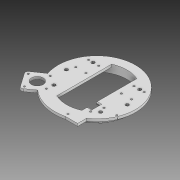
# Autodesk Inventor part: SwivelMount
Saved by Autodesk Inventor 2020 (Build 240168000, 168)
## iProperties
Created: 2020-09-15
Part Number: SwivelMount
Material: Generic
Document SubType Name: Modeling
Designer: DDeGo
Density: 1 g/cm^3
Appearance: Default
Author: DDeGo
Autodesk Inventor part; units mm, degrees
ref_plane "YZ Plane" through (0, 0, 0) normal (1, 0, 0) x (0, 1, 0)
ref_plane "XZ Plane" through (0, 0, 0) normal (0, 1, 0) x (-1, 0, 0)
ref_plane "XY Plane" through (0, 0, 0) normal (0, 0, 1) x (1, 0, 0)
sketch "Sketch1" plane through (0, 0, 0) normal (1, 0, 0) x (0, 1, 0)
  line L0 (0, 0) -> (0, -59.4) construction
  line L1 (0, -59.4) -> (7.5, -59.4)
  line L2 (7.5, -59.4) -> (7.5, -66.4) construction
  line L3 (7.5, -66.4) -> (5, -66.4)
  line L4 (5, -66.4) -> (5, -63.4)
  line L5 (5, -63.4) -> (0, -63.4)
  line L6 (0, -63.4) -> (0, -59.4)
  line L7 (0, 0) -> (7.5, 0) construction
  line L8 (7.5, 0) -> (7.5, -66.4) construction
  line L9 (7.5, -66.4) -> (11, -66.4)
  line L10 (11, -66.4) -> (11, -76)
  line L11 (11, -76) -> (16, -76)
  line L12 (16, -76) -> (16, -59.4)
  line L13 (16, -59.4) -> (7.5, -59.4)
  dimension "d0" = 63.4
  dimension "d1" = 4
  dimension "d2" = 2.5
  dimension "d3" = 3
  dimension "d4" = 5
  dimension "d6" = 6
  dimension "d7" = 5
  dimension "d8" = 76
  constraints: 28 end point, 10 perpendicular, 2 horizontal, 1 collinear, 1 point on line, 1 vertical
  measures "d0" distance from line of L0.start L5
  measures "d1" distance between parallel lines of L1 L5
  measures "d2" distance between parallel lines of L2 L4
  measures "d3" distance of L3.end L4.end
  measures "d4" distance of L4.end L5.end
  measures "d6" distance between parallel lines of L4 L10
  measures "d7" distance of L10.end L11.end
  measures "d8" distance between parallel lines of L7 L11
revolve "Revolution1" add sketch "Sketch1" angle 360 about axis through (0, 0, 0) along (0, 1, 0)
sketch "Sketch2" plane through (0, 16, 0) normal (0, 1, 0) x (1, 0, 0)
  line L0 (-24.75, -59.4) -> (24.75, -59.4)
  line L1 (24.75, -59.4) -> (24.75, 59.4)
  line L2 (24.75, 59.4) -> (-24.75, 59.4)
  line L3 (-24.75, 59.4) -> (-24.75, -59.4)
  line L4 (-24.75, -59.4) -> (24.75, 59.4) construction
  line L5 (24.75, -59.4) -> (-24.75, 59.4) construction
  circle A0 centre (0, 0) radius 59.4 projected
  point P0 (24.75, -53.9981)
  point P1 (24.75, 53.9981)
  point P2 (-24.75, -53.9981)
  point P3 (-24.75, 53.9981)
  dimension "d9" = 49.5
  constraints: 12 end point, 2 midpoint, 2 parallel, 1 horizontal, 1 perpendicular, 1 tangent
  measures "d9" distance of L1.end L2.end
extrude "Extrusion1" add sketch "Sketch2" against normal blind 5 contours A0 L3 | L1 A0
sketch "Sketch3" plane through (0, 16, 0) normal (0, 1, 0) x (1, 0, 0)
  line L0 (-44.75, 26) -> (0, 26) construction
  line L1 (24.75, 53.9981) -> (24.75, -53.9981) projected
  line L2 (-24.75, -53.9981) -> (-24.75, 53.9981) projected
  line L3 (-34.75, 13.5) -> (-54.75, 13.5) construction
  line L4 (-54.75, 13.5) -> (-54.75, 38.5) construction
  line L5 (-54.75, 38.5) -> (-34.75, 38.5) construction
  line L6 (-34.75, 38.5) -> (-34.75, 13.5) construction
  line L7 (-34.75, 13.5) -> (-54.75, 38.5) construction
  line L8 (-54.75, 13.5) -> (-34.75, 38.5) construction
  line L9 (0, 0) -> (0, 26) construction
  circle A0 centre (-54.75, 13.5) radius 1.75
  circle A1 centre (-54.75, 38.5) radius 1.75
  circle A2 centre (-34.75, 38.5) radius 1.75
  circle A3 centre (-34.75, 13.5) radius 1.75
  line L10 (34.75, 13.5) -> (54.75, 13.5) construction
  line L11 (54.75, 13.5) -> (54.75, 38.5) construction
  line L12 (54.75, 38.5) -> (34.75, 38.5) construction
  line L13 (34.75, 38.5) -> (34.75, 13.5) construction
  line L14 (34.75, 13.5) -> (54.75, 38.5) construction
  line L15 (54.75, 13.5) -> (34.75, 38.5) construction
  circle A4 centre (54.75, 13.5) radius 1.75
  circle A5 centre (54.75, 38.5) radius 1.75
  circle A6 centre (34.75, 38.5) radius 1.75
  circle A7 centre (34.75, 13.5) radius 1.75
  point P0 (44.75, 26)
  dimension "d12" = 26
  dimension "d14" = 20
  dimension "d15" = 25
  dimension "d16" = 20
  dimension "d17" = 3.5
  constraints: 28 end point, 9 symmetric about line, 8 centre point, 8 coincident, 4 midpoint, 3 equal radius, 2 horizontal, 2 parallel, 1 perpendicular, 1 vertical, 4 other
  measures "d12" distance from line of L9.start L0
  measures "d14" distance from line of L0.start L2
  measures "d15" distance of L3.end L4.end
  measures "d16" distance of L4.end L5.end
  measures "d17" diameter of A0
extrude "Extrusion2" cut sketch "Sketch3" against normal through all
sketch "Sketch4" plane through (0, 16, 0) normal (0, 1, 0) x (1, 0, 0)
  circle A0 centre (0, 0) radius 76 projected
  line L0 (25, -131.7705) -> (-25, -131.7705)
  line L1 (-25, -131.7705) -> (-25, -71.7705)
  line L2 (-25, -71.7705) -> (25, -71.7705) construction
  line L3 (25, -71.7705) -> (25, -131.7705)
  line L4 (25, -131.7705) -> (-25, -71.7705) construction
  line L5 (-25, -131.7705) -> (25, -71.7705) construction
  line L6 (0, -101.7705) -> (0, 0) construction
  point P0 (0, 0)
  dimension "d20" = 60
  dimension "d21" = 50
  constraints: 14 end point, 2 midpoint, 2 parallel, 1 horizontal, 1 perpendicular, 1 vertical, 2 other
  measures "d20" distance of L0.end L1.end
  measures "d21" distance of L0.start L0.end
extrude "Extrusion3" add sketch "Sketch4" against normal up to surface (5 mm away) contours A0 L3 L0 L1
sketch "Sketch5" plane through (-25, 16, 131.7705) normal (0, 1, 0) x (1, 0, 0)
  line L0 (-38.6517, 112.8373) -> (-14.5615, 78.433)
  line L1 (-14.5615, 78.433) -> (-44.8701, 57.2106)
  line L2 (-51.8337, 58.4385) -> (-70.1882, 84.6514)
  line L3 (-68.9603, 91.615) -> (-38.6517, 112.8373)
  line L4 (-22.2215, 79.7836) -> (-40.0023, 105.1773) construction
  line L5 (-40.0023, 105.1773) -> (-65.3961, 87.3965) construction
  line L6 (-65.3961, 87.3965) -> (-47.6152, 62.0028) construction
  line L7 (-47.6152, 62.0028) -> (-22.2215, 79.7836) construction
  arc A0 (50, 60) -> (0, 60) centre (25, 131.7705) ccw projected
  line L8 (-65.3961, 87.3965) -> (-22.2215, 79.7836) construction
  circle A1 centre (25, 131.7705) radius 63.4 projected
  line L9 (-43.8088, 83.59) -> (-26.9342, 95.4057) construction
  line L10 (-26.9342, 95.4057) -> (25, 131.7705) construction
  circle A2 centre (-40.0023, 105.1773) radius 1.75
  circle A3 centre (-65.3961, 87.3965) radius 1.75
  circle A4 centre (-43.8088, 83.59) radius 11.5
  circle A5 centre (-47.6152, 62.0028) radius 1.75
  circle A6 centre (-22.2215, 79.7836) radius 1.75
  line L11 (25, 131.7705) -> (25, 92.5102) construction
  arc A7 (-68.9603, 91.615) -> (-70.1882, 84.6514) centre (-66.0924, 87.5193) ccw
  arc A8 (-51.8337, 58.4385) -> (-44.8701, 57.2106) centre (-47.738, 61.3064) ccw
  point P0 (-48.9659, 54.3427)
  point P1 (-73.0561, 88.7471)
  point P2 (-22.7866, 72.6736)
  point P3 (-46.8769, 107.078)
  dimension "d24" = 20.6
  dimension "d25" = 31
  dimension "d26" = 42
  dimension "d29" = 3.5
  dimension "d30" = 23
  dimension "d31" = 55
  dimension "d37" = 5
  dimension "d38" = 84
  constraints: 24 end point, 7 centre point, 5 coincident, 4 equal radius, 4 parallel, 4 perpendicular, 4 point on circle, 4 point on line, 4 tangent, 1 collinear, 1 midpoint, 1 vertical, 5 other
  measures "d24" distance of L9.start L9.end
  measures "d25" distance of L5.end L6.end
  measures "d26" distance of point (-48.966, 54.343) point (-73.056, 88.747)
  measures "d29" diameter of A6
  measures "d30" diameter of A4
  measures "d31" angle of L10 L11
  measures "d37" radius of A7
  measures "d38" distance of point (25, 131.77) A4.centre
extrude "Extrusion4" add sketch "Sketch5" against normal up to surface (5 mm away) contours L0 A1 L1 A0 A4 L3 | L0 A1 | A0 A4 L1 A8 L2 A7 L3 | A4 A0 | A0 A4 | A2 | A3 | A5 | A6 picked at (-26.2496, 94.9188)
extrude "Extrusion5" cut sketch "Sketch5" against normal through all contours A4 A0 | A0 A4 | A2 | A3 | A5 | A6
sketch "Sketch6" plane through (-25, 11, 131.7705) normal (0, -1, 0) x (1, 0, 0)
  circle A0 centre (-65.3961, -87.3965) radius 1.75 projected
  circle A1 centre (-65.3961, -87.3965) radius 3
  circle A2 centre (-47.6152, -62.0028) radius 1.75 projected
  circle A3 centre (-47.6152, -62.0028) radius 3
  circle A4 centre (-22.2215, -79.7836) radius 1.75 projected
  circle A5 centre (-22.2215, -79.7836) radius 3
  circle A6 centre (-40.0023, -105.1773) radius 1.75 projected
  circle A7 centre (-40.0023, -105.1773) radius 3
  point P0 (25, -131.7705)
  dimension "d34" = 6
  constraints: 4 centre point, 4 coincident, 3 equal radius
  measures "d34" diameter of A1
extrude "Extrusion6" cut sketch "Sketch6" against normal blind 3 contours A0 | A1 | A2 | A3 | A4 | A5 | A6 | A7
ref_plane "Work Plane1" through (38.75, 16, -53.9981) normal (-1, 0, 0) x (0, 0, 1)
sketch "Sketch7" plane through (38.75, 16, -53.9981) normal (-1, 0, 0) x (0, 0, 1)
  line L0 (13.7481, 0) -> (17.2481, 0) projected
  line L1 (38.7481, 0) -> (42.2481, 0) projected
  line L2 (15.4981, 0) -> (27.9981, 40) construction
  line L3 (27.9981, 40) -> (40.4981, 0) construction
  line L4 (27.9981, 40) -> (109.9356, 21.5) construction
  line L5 (94.4356, 37) -> (125.4356, 37) construction
  line L6 (125.4356, 37) -> (125.4356, 6) construction
  line L7 (125.4356, 6) -> (94.4356, 6) construction
  line L8 (94.4356, 6) -> (94.4356, 37) construction
  line L9 (94.4356, 37) -> (125.4356, 6) construction
  line L10 (125.4356, 37) -> (94.4356, 6) construction
  circle A0 centre (109.9356, 21.5) radius 11.5
  circle A1 centre (125.4356, 37) radius 1.75
  circle A2 centre (125.4356, 6) radius 1.75
  circle A3 centre (94.4356, 6) radius 1.75
  circle A4 centre (94.4356, 37) radius 1.75
  line L11 (88.4356, 0) -> (131.4356, 0)
  line L12 (131.4356, 0) -> (131.4356, 43)
  line L13 (131.4356, 43) -> (88.4356, 43)
  line L14 (88.4356, 43) -> (88.4356, 0)
  line L15 (88.4356, 0) -> (131.4356, 43) construction
  line L16 (131.4356, 0) -> (88.4356, 43) construction
  line L17 (0, 0) -> (107.9962, 0) projected
  point P0 (53.9981, -16)
  dimension "d40" = 84
  dimension "d41" = 23
  dimension "d42" = 3.5
  dimension "d43" = 31
  dimension "d44" = 31
  dimension "d46" = 40
  dimension "d47" = 43
  dimension "d84" = 81.9375
  constraints: 30 end point, 6 midpoint, 5 centre point, 5 coincident, 4 parallel, 3 equal radius, 2 horizontal, 2 perpendicular, 1 equal length, 1 point on line, 2 other
  measures "d40" distance of L2.end L4.end
  measures "d41" diameter of A0
  measures "d42" diameter of A4
  measures "d43" distance of L5.start L5.end
  measures "d44" distance of L7.end L5.start
  measures "d46" distance from line of L1 L2.end
  measures "d47" distance of L11.end L12.end
  measures "d84" horizontal distance of L4.end L2.end
extrude "Extrusion7" add sketch "Sketch7" against normal blind 4
sketch "Sketch8" plane through (38.75, 16, 65.3792) normal (0, -1, 0) x (1, 0, 0)
  arc A0 (-110.6269, -40.6867) -> (4, -2.5426) centre (-38.75, -65.3792) ccw projected
  line L0 (0, 12.0583) -> (4, 12.0583) projected
  line L1 (4, -2.5426) -> (4, 12.0583)
  line L2 (4, 12.0583) -> (-13.75, 12.0583)
  line L3 (-13.75, 66.3913) -> (-13.75, 6.3913) projected
  arc A1 (0, 0) -> (-13.75, 6.3913) centre (-38.75, -65.3792) ccw projected
  line L4 (-13.75, 12.0583) -> (-13.75, 6.3913)
  arc A2 (4, -2.5426) -> (-13.75, 6.3913) centre (-38.75, -65.3792) ccw
  arc A3 (-110.6269, -40.6867) -> (-13.75, 6.3913) centre (-38.75, -65.3792) ccw projected
  constraints: 6 end point, 2 perpendicular, 2 point on circle, 1 centre point, 1 concentric, 1 point on line, 1 vertical
extrude "Extrusion8" add sketch "Sketch8" along normal up to surface (5 mm away)
sketch "Sketch9" plane through (25, 16, 77.4375) normal (0, 0, 1) x (1, 0, 0)
  line L0 (17.75, 43) -> (17.75, -5) projected
  line L1 (13.75, 0) -> (13.75, 43) construction
  line L2 (17.75, 43) -> (13.75, 43)
  line L3 (13.75, 43) -> (-6.25, 0)
  line L4 (0, -5) -> (0.4629, 0) construction
  line L5 (-6.25, 0) -> (0, -5)
  line L6 (0, -5) -> (17.75, -5) projected
  line L7 (0, -5) -> (17.75, -5)
  line L8 (17.75, -5) -> (17.75, 43)
  line L9 (13.75, 0) -> (0, 0) construction
  point P0 (-25, -16)
  dimension "d52" = 20
  constraints: 12 end point, 2 perpendicular, 2 point on line, 1 collinear
  measures "d52" distance from line of L1 L3.end
extrude "Extrusion9" add sketch "Sketch9" along normal blind 3
sketch "Sketch10" plane through (38.75, 16, 34.4375) normal (0, 0, -1) x (-1, 0, 0)
  line L0 (0, 43) -> (-4, 43) projected
  line L1 (-4, 43) -> (-28.3595, 0)
  line L2 (-37.25, 0) -> (114.75, 0) projected
  line L3 (0, 43) -> (0, 0) projected
  line L4 (-28.3595, 0) -> (0, 0)
  line L5 (0, 0) -> (0, 43)
  line L6 (0, 43) -> (-4, 43)
  point P0 (38.75, -16)
  point P1 (110.6269, 0)
  point P2 (-4, 0)
  dimension "d85" = 28.3595
  constraints: 8 end point, 2 perpendicular, 1 horizontal, 1 point on line
  measures "d85" distance from line of L1.end L3
extrude "Extrusion10" add sketch "Sketch10" along normal blind 3
sketch "Sketch11" plane through (-25, 16, 131.7705) normal (0, 1, 0) x (1, 0, 0)
  line L0 (49.75, 77.7723) -> (49.75, 185.7686) projected
  line L1 (49.75, 89.7723) -> (58.75, 89.7723)
  line L2 (58.75, 89.7723) -> (58.75, 105.7723)
  line L3 (58.75, 105.7723) -> (49.75, 105.7723)
  line L4 (49.75, 105.7723) -> (49.75, 89.7723)
  point P0 (25, 131.7705)
  dimension "d57" = 9
  dimension "d58" = 12
  dimension "d59" = 16
  constraints: 8 end point, 2 parallel, 1 horizontal, 1 perpendicular, 1 point on line
  measures "d57" distance between parallel lines of L0 L2
  measures "d58" distance from line of L0.start L1
  measures "d59" distance of L1.end L2.end
extrude "Extrusion11" cut sketch "Sketch11" against normal through all
fillet "Fillet1" radius 2 4 edges at (29.25, 11, 41.9981) (29.25, 11, 25.9981) (29.25, 16, 41.9981) (29.25, 16, 25.9981)
sketch "Sketch12" plane through (-25, 16, 131.7705) normal (0, 1, 0) x (1, 0, 0)
  line L0 (43.75, 51.333) -> (43.75, 54.333) projected
  circle A0 centre (25, 131.7705) radius 82.5939
  line L1 (0, 60) -> (0, 0) projected
  arc A1 (-22.7866, 72.6736) -> (0, 60) centre (25, 131.7705) ccw projected
  line L2 (-44.8701, 57.2106) -> (-22.7866, 72.6736) projected
  point P0 (-28.3884, 68.7512)
  point P1 (0, 53.051)
  constraints: 1 coincident, 3 other
extrude "Extrusion12" add sketch "Sketch12" against normal up to surface (5 mm away) contours A0 L2 A1 L1 picked at (-12.6124, 60.8804)
sketch "Sketch13" plane through (-25, 16, 131.7705) normal (0, 1, 0) x (1, 0, 0)
  arc A0 (-28.3884, 68.7512) -> (0, 53.051) centre (25, 131.7705) ccw projected
  circle A1 centre (25, 131.7705) radius 82.5939
  circle A2 centre (-29.75, 145.2705) radius 1.75 projected
  circle A3 centre (79.75, 170.2705) radius 1.75 projected
  circle A4 centre (59.75, 145.2705) radius 1.75 projected
  circle A5 centre (79.75, 145.2705) radius 1.75 projected
  circle A6 centre (-9.75, 145.2705) radius 1.75 projected
  circle A7 centre (-29.75, 170.2705) radius 1.75 projected
  circle A8 centre (-9.75, 170.2705) radius 1.75 projected
  circle A9 centre (59.75, 170.2705) radius 1.75 projected
  circle A10 centre (-40.0023, 105.1773) radius 1.75 projected
  circle A11 centre (-65.3961, 87.3965) radius 1.75 projected
  circle A12 centre (-43.8088, 83.59) radius 11.5 projected
  circle A13 centre (-47.6152, 62.0028) radius 1.75 projected
  circle A14 centre (-22.2215, 79.7836) radius 1.75 projected
  line L0 (92.1095, 97.333) -> (67.75, 97.333) projected
  line L1 (67.75, 97.333) -> (67.75, 68.9339) projected
  arc A15 (67.75, 68.9339) -> (-46.8769, 107.078) centre (25, 131.7705) ccw projected
  line L2 (-46.8769, 107.078) -> (-68.9603, 91.615) projected
  arc A16 (-68.9603, 91.615) -> (-70.1882, 84.6514) centre (-66.0924, 87.5193) ccw projected
  line L3 (-70.1882, 84.6514) -> (-51.8337, 58.4385) projected
  arc A17 (-51.8337, 58.4385) -> (-44.8701, 57.2106) centre (-47.738, 61.3064) ccw projected
  line L4 (-44.8701, 57.2106) -> (-28.3884, 68.7512) projected
  arc A18 (-28.3884, 68.7512) -> (0, 53.051) centre (25, 131.7705) ccw projected
  line L5 (0, 53.051) -> (0, 0) projected
  line L6 (0, 0) -> (50, 0) projected
  line L7 (50, 0) -> (50, 51.333) projected
  line L8 (50, 51.333) -> (43.75, 51.333) projected
  line L9 (43.75, 51.333) -> (43.75, 54.333) projected
  line L10 (63.75, 54.333) -> (43.75, 54.333) projected
  line L11 (63.75, 54.333) -> (63.75, 100.333) projected
  line L12 (63.75, 100.333) -> (92.1095, 100.333) projected
  line L13 (92.1095, 100.333) -> (92.1095, 97.333) projected
  line L14 (58.75, 107.7723) -> (49.75, 107.7723) projected
  line L15 (58.75, 107.7723) -> (58.75, 87.7723) projected
  line L16 (49.75, 87.7723) -> (58.75, 87.7723) projected
  line L17 (49.75, 87.7723) -> (49.75, 77.7723) projected
  arc A19 (0.25, 77.7723) -> (49.75, 77.7723) centre (25, 131.7705) ccw projected
  line L18 (0.25, 77.7723) -> (0.25, 185.7686) projected
  arc A20 (49.75, 185.7686) -> (0.25, 185.7686) centre (25, 131.7705) ccw projected
  line L19 (49.75, 185.7686) -> (49.75, 107.7723) projected
  point P0 (43.75, 51.333)
  point P1 (0, 53.051)
  constraints: 1 coincident, 3 other
extrude "Extrusion13" cut sketch "Sketch13" against normal through all contours A1 L8 L7 L6 L5
sketch "Sketch14" plane through (0, 11, 0) normal (0, -1, 0) x (1, 0, 0)
  circle A0 centre (-34.75, -13.5) radius 1.75 projected
  line L0 (-34.75, -16.8486) -> (-37.65, -15.1743)
  line L1 (-37.65, -15.1743) -> (-37.65, -11.8257)
  line L2 (-37.65, -11.8257) -> (-34.75, -10.1514)
  line L3 (-34.75, -10.1514) -> (-31.85, -11.8257)
  line L4 (-31.85, -11.8257) -> (-31.85, -15.1743)
  line L5 (-31.85, -15.1743) -> (-34.75, -16.8486)
  circle A1 centre (-54.75, -13.5) radius 1.75 projected
  line L6 (-54.75, -16.8486) -> (-57.65, -15.1743)
  line L7 (-57.65, -15.1743) -> (-57.65, -11.8257)
  line L8 (-57.65, -11.8257) -> (-54.75, -10.1514)
  line L9 (-54.75, -10.1514) -> (-51.85, -11.8257)
  line L10 (-51.85, -11.8257) -> (-51.85, -15.1743)
  line L11 (-51.85, -15.1743) -> (-54.75, -16.8486)
  circle A2 centre (-34.75, -38.5) radius 1.75 projected
  line L12 (-34.75, -35.1514) -> (-31.85, -36.8257)
  line L13 (-31.85, -36.8257) -> (-31.85, -40.1743)
  line L14 (-31.85, -40.1743) -> (-34.75, -41.8486)
  line L15 (-34.75, -41.8486) -> (-37.65, -40.1743)
  line L16 (-37.65, -40.1743) -> (-37.65, -36.8257)
  line L17 (-37.65, -36.8257) -> (-34.75, -35.1514)
  circle A3 centre (-54.75, -38.5) radius 1.75 projected
  line L18 (-53.0757, -41.4) -> (-56.4243, -41.4)
  line L19 (-56.4243, -41.4) -> (-58.0986, -38.5)
  line L20 (-58.0986, -38.5) -> (-56.4243, -35.6)
  line L21 (-56.4243, -35.6) -> (-53.0757, -35.6)
  line L22 (-53.0757, -35.6) -> (-51.4014, -38.5)
  line L23 (-51.4014, -38.5) -> (-53.0757, -41.4)
  circle A4 centre (34.75, -13.5) radius 1.75 projected
  line L24 (34.75, -16.8486) -> (31.85, -15.1743)
  line L25 (31.85, -15.1743) -> (31.85, -11.8257)
  line L26 (31.85, -11.8257) -> (34.75, -10.1514)
  line L27 (34.75, -10.1514) -> (37.65, -11.8257)
  line L28 (37.65, -11.8257) -> (37.65, -15.1743)
  line L29 (37.65, -15.1743) -> (34.75, -16.8486)
  circle A5 centre (34.75, -38.5) radius 1.75 projected
  line L30 (34.75, -35.1514) -> (37.65, -36.8257)
  line L31 (37.65, -36.8257) -> (37.65, -40.1743)
  line L32 (37.65, -40.1743) -> (34.75, -41.8486)
  line L33 (34.75, -41.8486) -> (31.85, -40.1743)
  line L34 (31.85, -40.1743) -> (31.85, -36.8257)
  line L35 (31.85, -36.8257) -> (34.75, -35.1514)
  circle A6 centre (54.75, -13.5) radius 1.75 projected
  line L36 (54.75, -10.1514) -> (57.65, -11.8257)
  line L37 (57.65, -11.8257) -> (57.65, -15.1743)
  line L38 (57.65, -15.1743) -> (54.75, -16.8486)
  line L39 (54.75, -16.8486) -> (51.85, -15.1743)
  line L40 (51.85, -15.1743) -> (51.85, -11.8257)
  line L41 (51.85, -11.8257) -> (54.75, -10.1514)
  arc A7 (53.3431, -39.5408) -> (55.2535, -36.824) centre (54.75, -38.5) ccw projected
  line L42 (53.0757, -41.4) -> (51.4014, -38.5)
  line L43 (51.4014, -38.5) -> (53.0757, -35.6)
  line L44 (53.0757, -35.6) -> (56.4243, -35.6)
  line L45 (56.4243, -35.6) -> (58.0986, -38.5)
  line L46 (58.0986, -38.5) -> (56.4243, -41.4)
  line L47 (56.4243, -41.4) -> (53.0757, -41.4)
  point P0 (0, 0)
  dimension "d67" = 5.8
  constraints: 96 end point, 8 coincident, 7 equal length, 6 vertical, 2 horizontal, 104 other
  measures "d67" distance between parallel lines of L4 L1
extrude "Extrusion14" cut sketch "Sketch14" along normal blind 15 and the other way blind 2.5 contours A0 | L0 L1 L2 L3 L4 L5 | A1 | L6 L7 L8 L9 L10 L11 | A2 | L12 L13 L14 L15 L16 L17 | A3 | L18 L19 L20 L21 L22 L23 | A4 | L24 L25 L26 L27 L28 L29 | A5 | L30 L31 L32 L33 L34 L35 | A6 | L36 L37 L38 L39 L40 L41 | L42 L43 L44 L45 L46 L47
sketch "Sketch15" plane through (0, 0, 0) normal (0, -1, 0) x (1, 0, 0)
  line L0 (0, 0) -> (0, 59.4) construction
  arc A0 (24.75, 53.9981) -> (-24.75, 53.9981) centre (0, 0) ccw construction
  line L1 (0, 0) -> (-59.4, 0) construction
  line L2 (0, 0) -> (-45.503, -38.1816) construction
  arc A1 (-57.3891, -15.325) -> (57.3891, -15.325) centre (0, 0) ccw construction
  line L3 (0, 0) -> (-45.503, 38.1816) construction
  circle A2 centre (-45.8861, 38.503) radius 3.5 construction
  circle A3 centre (0, 0) radius 63.4 projected
  circle A4 centre (-59.9, 0) radius 3.5 construction
  circle A5 centre (-45.8861, -38.503) radius 3.5 construction
  circle A6 centre (-45.8861, 38.503) radius 1.75
  circle A7 centre (-45.8861, 38.503) radius 4.5
  circle A8 centre (-59.9, 0) radius 4.5
  circle A9 centre (-59.9, 0) radius 1.75
  circle A10 centre (-45.8861, -38.503) radius 1.75
  circle A11 centre (-45.8861, -38.503) radius 4.5
  circle A12 centre (45.8861, 38.503) radius 3.5 construction
  circle A13 centre (59.9, 0) radius 3.5 construction
  circle A14 centre (45.8861, -38.503) radius 3.5 construction
  circle A15 centre (45.8861, 38.503) radius 1.75
  circle A16 centre (45.8861, 38.503) radius 4.5
  circle A17 centre (59.9, 0) radius 4.5
  circle A18 centre (59.9, 0) radius 1.75
  circle A19 centre (45.8861, -38.503) radius 1.75
  circle A20 centre (45.8861, -38.503) radius 4.5
  point P0 (59.4, 0)
  point P1 (45.503, -38.1816)
  point P2 (45.503, 38.1816)
  point P3 (50.386, 38.4813)
  point P4 (46.6461, 42.9383)
  point P5 (63.3332, 2.9091)
  point P6 (63.3332, -2.9091)
  point P7 (46.6461, -42.9383)
  point P8 (50.386, -38.4813)
  point P9 (-50.386, -38.4813)
  point P10 (-46.6461, -42.9383)
  point P11 (-63.3332, 2.9091)
  point P12 (-63.3332, -2.9091)
  point P13 (-50.386, 38.4813)
  point P14 (-46.6461, 42.9383)
  dimension "d72" = 40
  dimension "d73" = 40
  dimension "d74" = 7
  dimension "d75" = 9
  dimension "d76" = 3.5
  constraints: 18 centre point, 12 coincident, 12 symmetric about line, 8 end point, 6 equal radius, 3 point on line, 3 tangent, 2 point on circle, 1 horizontal, 1 vertical, 9 other
  measures "d72" angle of L3 L1
  measures "d73" angle of L2 L1
  measures "d74" diameter of A2
  measures "d75" diameter of A11
  measures "d76" diameter of A10
extrude "Extrusion15" add sketch "Sketch15" against normal up to surface (11 mm away) contours A3 A17 | A16 A3 | A3 A16 | A3 A20 | A7 A3 | A3 A11 | A8 A3 | A6 | A9 | A10 | A18 | A19 picked at (62.3698, 2.2508) picked at (46.8937, -41.5565) picked at (-46.8937, 41.5565) picked at (-46.8937, -41.5565) picked at (-62.6452, 1.6799)
extrude "Extrusion16" cut sketch "Sketch15" against normal up to surface (16 mm away) contours A6 | A9 | A10 | A15 | A18 | A19
sketch "Sketch16" plane through (18.75, 16, 77.4375) normal (0, 1, 0) x (1, 0, 0)
  circle A0 centre (-64.6361, 115.9405) radius 1.75 projected
  line L0 (-61.7361, 117.6148) -> (-61.7361, 114.2661)
  line L1 (-61.7361, 114.2661) -> (-64.6361, 112.5918)
  line L2 (-64.6361, 112.5918) -> (-67.5361, 114.2661)
  line L3 (-67.5361, 114.2661) -> (-67.5361, 117.6148)
  line L4 (-67.5361, 117.6148) -> (-64.6361, 119.2891)
  line L5 (-64.6361, 119.2891) -> (-61.7361, 117.6148)
  circle A1 centre (-78.65, 77.4375) radius 1.75 projected
  line L6 (-78.65, 80.7861) -> (-75.75, 79.1118)
  line L7 (-75.75, 79.1118) -> (-75.75, 75.7632)
  line L8 (-75.75, 75.7632) -> (-78.65, 74.0888)
  line L9 (-78.65, 74.0888) -> (-81.55, 75.7632)
  line L10 (-81.55, 75.7632) -> (-81.55, 79.1118)
  line L11 (-81.55, 79.1118) -> (-78.65, 80.7861)
  circle A2 centre (-64.6361, 38.9345) radius 1.75 projected
  line L12 (-64.6361, 35.5859) -> (-67.5361, 37.2602)
  line L13 (-67.5361, 37.2602) -> (-67.5361, 40.6088)
  line L14 (-67.5361, 40.6088) -> (-64.6361, 42.2831)
  line L15 (-64.6361, 42.2831) -> (-61.7361, 40.6088)
  line L16 (-61.7361, 40.6088) -> (-61.7361, 37.2602)
  line L17 (-61.7361, 37.2602) -> (-64.6361, 35.5859)
  circle A3 centre (27.1361, 38.9345) radius 1.75 projected
  line L18 (30.0361, 37.2602) -> (27.1361, 35.5859)
  line L19 (27.1361, 35.5859) -> (24.2361, 37.2602)
  line L20 (24.2361, 37.2602) -> (24.2361, 40.6088)
  line L21 (24.2361, 40.6088) -> (27.1361, 42.2831)
  line L22 (27.1361, 42.2831) -> (30.0361, 40.6088)
  line L23 (30.0361, 40.6088) -> (30.0361, 37.2602)
  circle A4 centre (41.15, 77.4375) radius 1.75 projected
  line L24 (41.15, 80.7861) -> (44.05, 79.1118)
  line L25 (44.05, 79.1118) -> (44.05, 75.7632)
  line L26 (44.05, 75.7632) -> (41.15, 74.0888)
  line L27 (41.15, 74.0888) -> (38.25, 75.7632)
  line L28 (38.25, 75.7632) -> (38.25, 79.1118)
  line L29 (38.25, 79.1118) -> (41.15, 80.7861)
  circle A5 centre (27.1361, 115.9405) radius 1.75 projected
  line L30 (27.1361, 112.5918) -> (24.2361, 114.2661)
  line L31 (24.2361, 114.2661) -> (24.2361, 117.6148)
  line L32 (24.2361, 117.6148) -> (27.1361, 119.2891)
  line L33 (27.1361, 119.2891) -> (30.0361, 117.6148)
  line L34 (30.0361, 117.6148) -> (30.0361, 114.2661)
  line L35 (30.0361, 114.2661) -> (27.1361, 112.5918)
  point P0 (-18.75, 77.4375)
  dimension "d81" = 5.8
  constraints: 72 end point, 6 coincident, 6 vertical, 5 equal length, 78 other
  measures "d81" distance between parallel lines of L3 L0
extrude "Extrusion17" cut sketch "Sketch16" against normal blind 5
sketch "Sketch17" plane through (38.75, 16, 31.4375) normal (0, 0, -1) x (-1, 0, 0)
  line L0 (-37.25, 0) -> (114.75, 0) projected
  line L1 (-36.9704, 60.3462) -> (31.4894, 60.3462)
  line L2 (31.4894, 60.3462) -> (31.4894, 0)
  line L3 (31.4894, 0) -> (-36.9704, 0)
  line L4 (-36.9704, 0) -> (-36.9704, 60.3462)
  point P0 (38.75, -16)
  point P1 (110.6269, 0)
  point P2 (-4, 0)
  constraints: 8 end point, 2 parallel, 1 horizontal, 1 perpendicular, 1 point on line
extrude "Extrusion18" cut sketch "Sketch17" against normal through all
sketch "Sketch18" plane through (42.75, 16, 80.4375) normal (0, 1, 0) x (1, 0, 0)
  circle A0 centre (-25.5, 6.5) radius 1.75
  circle A1 centre (-7.5, 33) radius 1.75
  line L0 (0, 17.6009) -> (0, 0) projected
  line L1 (0, 0) -> (-24, 0) projected
  circle A2 centre (24.5, 52.5) radius 1.75
  circle A3 centre (-0.5, 52.5) radius 1.75
  line L2 (24.5, 52.5) -> (-0.5, 52.5) construction
  point P0 (-42.75, 80.4375)
  dimension "d97" = 25.5
  dimension "d98" = 6.5
  dimension "d99" = 18
  dimension "d100" = 26.5
  dimension "d101" = 7
  dimension "d102" = 19.5
  dimension "d103" = 25
  dimension "d104" = 3.5
  constraints: 4 centre point, 3 equal radius, 2 end point, 1 horizontal
  measures "d97" distance from line of A0.centre L0
  measures "d98" distance from line of A0.centre L1
  measures "d99" horizontal distance of A0.centre A1.centre
  measures "d100" vertical distance of A0.centre A1.centre
  measures "d101" horizontal distance of A1.centre L2.end
  measures "d102" vertical distance of A1.centre L2.end
  measures "d103" distance of L2.start L2.end
  measures "d104" diameter of A0
extrude "Extrusion19" cut sketch "Sketch18" against normal up to surface (5 mm away)
sketch "Sketch19" plane through (0, 11, 0) normal (0, -1, 0) x (1, 0, 0)
  circle A0 centre (17.25, 73.9375) radius 1.75 projected
  line L0 (17.25, 77.2861) -> (20.15, 75.6118)
  line L1 (20.15, 75.6118) -> (20.15, 72.2632)
  line L2 (20.15, 72.2632) -> (17.25, 70.5888)
  line L3 (17.25, 70.5888) -> (14.35, 72.2632)
  line L4 (14.35, 72.2632) -> (14.35, 75.6118)
  line L5 (14.35, 75.6118) -> (17.25, 77.2861)
  circle A1 centre (35.25, 47.4375) radius 1.75 projected
  line L6 (32.35, 49.1118) -> (35.25, 50.7861)
  line L7 (35.25, 50.7861) -> (38.15, 49.1118)
  line L8 (38.15, 49.1118) -> (38.15, 45.7632)
  line L9 (38.15, 45.7632) -> (35.25, 44.0888)
  line L10 (35.25, 44.0888) -> (32.35, 45.7632)
  line L11 (32.35, 45.7632) -> (32.35, 49.1118)
  circle A2 centre (67.25, 27.9375) radius 1.75 projected
  line L12 (67.25, 31.2861) -> (70.15, 29.6118)
  line L13 (70.15, 29.6118) -> (70.15, 26.2632)
  line L14 (70.15, 26.2632) -> (67.25, 24.5888)
  line L15 (67.25, 24.5888) -> (64.35, 26.2632)
  line L16 (64.35, 26.2632) -> (64.35, 29.6118)
  line L17 (64.35, 29.6118) -> (67.25, 31.2861)
  circle A3 centre (42.25, 27.9375) radius 1.75 projected
  line L18 (42.25, 31.2861) -> (45.15, 29.6118)
  line L19 (45.15, 29.6118) -> (45.15, 26.2632)
  line L20 (45.15, 26.2632) -> (42.25, 24.5888)
  line L21 (42.25, 24.5888) -> (39.35, 26.2632)
  line L22 (39.35, 26.2632) -> (39.35, 29.6118)
  line L23 (39.35, 29.6118) -> (42.25, 31.2861)
  point P0 (0, 0)
  dimension "d107" = 5.8
  constraints: 48 end point, 4 coincident, 4 vertical, 3 parallel, 52 other
  measures "d107" distance between parallel lines of L19 L22
extrude "Extrusion20" cut sketch "Sketch19" along normal blind 3 and the other way blind 2.5 contours A0 | L0 L1 L2 L3 L4 L5 | A1 | L6 L7 L8 L9 L10 L11 | A2 | L12 L13 L14 L15 L16 L17 | A3 | L18 L19 L20 L21 L22 L23
chamfer "Chamfer1" distance 2.5 angle 45 1 edges at (35.5034, 8, 47.6221)
equation "\"d73\" = d72"
body "Solid1"
